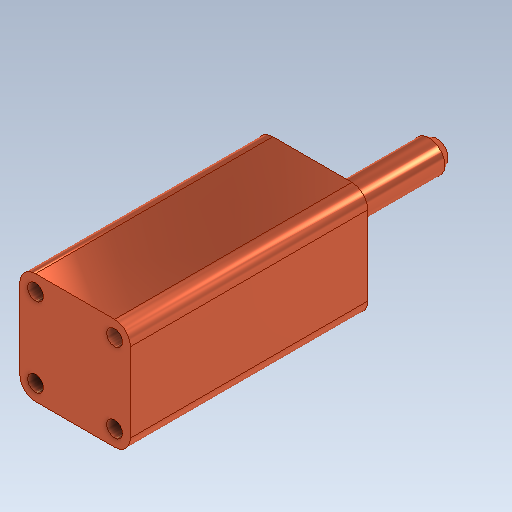
# Autodesk Inventor part: Silnik krokowy
Saved by Autodesk Inventor 2020 (Build 240168000, 168)
## iProperties
Created: 2021-10-14
Part Number: Silnik krokowy
Material: Ogólny
Document SubType Name: Modeling
Designer: Komputer
Density: 1 g/cm^3
Appearance: Gorący metal 1400F
Mass: 5.94241 g
Surface Area: 23.2204 cm^2
Volume: 5.94241 cm^3
Author: Komputer
Autodesk Inventor part; units mm, degrees
ref_plane "YZ Plane" through (0, 0, 0) normal (1, 0, 0) x (0, 1, 0)
ref_plane "XZ Plane" through (0, 0, 0) normal (0, 1, 0) x (-1, 0, 0)
ref_plane "XY Plane" through (0, 0, 0) normal (0, 0, 1) x (1, 0, 0)
sketch "Szkic1" plane through (0, 0, 0) normal (0, 0, 1) x (1, 0, 0)
  line L0 (7, -7) -> (-7, -7)
  line L1 (-7, -7) -> (-7, 7)
  line L2 (-7, 7) -> (7, 7)
  line L3 (7, 7) -> (7, -7)
  line L4 (7, -7) -> (-7, 7) construction
  line L5 (-7, -7) -> (7, 7) construction
  line L6 (0, 0) -> (-5.75, 0)
  line L7 (-7, 5.75) -> (-5, 5.75)
  line L8 (-5, 7) -> (-5, 5)
  line L9 (-5, 5) -> (5, 5)
  line L10 (5, 5) -> (5, -5)
  line L11 (5, -5) -> (-5, -5)
  line L12 (-5, -5) -> (-5, 5)
  circle A0 centre (-5, 5) radius 1
  circle A1 centre (5, 5) radius 1
  circle A2 centre (5, -5) radius 1
  circle A3 centre (-5, -5) radius 1
  circle A4 centre (0, 0) radius 5
  circle A5 centre (0, 0) radius 5.5
  circle A6 centre (0, 0) radius 2
  circle A7 centre (0, 0) radius 2.1
  dimension "d0" = 14
  dimension "d1" = 14
  dimension "d8" = 2
  dimension "d9" = 2
  dimension "d13" = 10
  dimension "d14" = 10
  dimension "d15" = 10
  dimension "d17" = 2
  dimension "d18" = 2
  dimension "d19" = 2
  dimension "d20" = 2
  dimension "d21" = 11
  dimension "d22" = 4
  dimension "d23" = 4.2
  constraints: 26 end point, 8 centre point, 8 coincident, 6 point on line, 3 perpendicular, 2 horizontal, 2 midpoint, 2 parallel
  measures "d0" distance of L1.end L2.end
  measures "d1" distance of L0.end L1.end
  measures "d8" distance of L7.start L7.end
  measures "d9" distance of L8.start L8.end
  measures "d13" distance of L8.end L9.end
  measures "d14" distance of L9.end L10.end
  measures "d15" distance of L10.end L11.end
  measures "d17" diameter of A0
  measures "d18" diameter of A1
  measures "d19" diameter of A2
  measures "d20" diameter of A3
  measures "d21" diameter of A5
  measures "d22" diameter of A6
  measures "d23" diameter of A7
extrude "Wyciągnięcie proste1" add sketch "Szkic1" along normal blind 30 contours L0 L1 L7 A0 L12 A5 A3 L11 A2 L10 A1 L9 L8 L2 L3 | L1 L2 L8 A0 L7 | A0 L9 A5 L12 | A5 L9 A4 L12 | L12 L6 A5 | A5 L9 | A6 | A7 | L12 A5 L6 | A4 L11 A5 L12 | A4 | L9 A5 L10 A4 | L9 A1 L10 A5 | A5 L11 A3 L12 | A4 L10 A5 L11 | L11 A5 | L10 A5 | A5 L10 A2 L11
sketch "Szkic2" plane through (0, 0, 0) normal (0, 0, -1) x (-1, 0, 0)
  line L0 (7, -7) -> (-7, -7)
  line L1 (-7, -7) -> (-7, 7)
  line L2 (-7, 7) -> (7, 7)
  line L3 (7, 7) -> (7, -7)
  line L4 (7, -7) -> (-7, 7) construction
  line L5 (-7, -7) -> (7, 7) construction
  line L6 (0, 0) -> (-5.75, 0)
  line L7 (-7, 5.75) -> (-5, 5.75)
  line L8 (-5, 7) -> (-5, 5)
  line L9 (-5, 5) -> (5, 5)
  line L10 (5, 5) -> (5, -5)
  line L11 (5, -5) -> (-5, -5)
  line L12 (-5, -5) -> (-5, 5)
  circle A0 centre (-5, 5) radius 1
  circle A1 centre (5, 5) radius 1
  circle A2 centre (5, -5) radius 1
  circle A3 centre (-5, -5) radius 1
  circle A4 centre (0, 0) radius 5
  circle A5 centre (0, 0) radius 5.5
  circle A6 centre (0, 0) radius 2
  circle A7 centre (0, 0) radius 2.1
  dimension "d26" = 14
  dimension "d27" = 14
  dimension "d28" = 2
  dimension "d29" = 2
  dimension "d30" = 10
  dimension "d31" = 10
  dimension "d32" = 10
  dimension "d33" = 2
  dimension "d34" = 2
  dimension "d35" = 2
  dimension "d36" = 2
  dimension "d37" = 11
  dimension "d38" = 4
  dimension "d39" = 4.2
  constraints: 26 end point, 8 centre point, 8 coincident, 6 point on line, 3 perpendicular, 2 horizontal, 2 midpoint, 2 parallel
  measures "d26" distance of L1.end L3.start
  measures "d27" distance of L0.end L1.end
  measures "d28" distance of L7.start L7.end
  measures "d29" distance of L8.start L12.end
  measures "d30" distance of L12.end L10.start
  measures "d31" distance of L10.start L11.start
  measures "d32" distance of L11.start L11.end
  measures "d33" diameter of A0
  measures "d34" diameter of A1
  measures "d35" diameter of A2
  measures "d36" diameter of A3
  measures "d37" diameter of A5
  measures "d38" diameter of A6
  measures "d39" diameter of A7
extrude "Wyciągnięcie proste2" add sketch "Szkic2" along normal blind 0.75 contours A6 | A7 | A4
fillet "Zaokrąglenie1" radius 2 4 edges at (-7, 7, 15) (7, 7, 15) (7, -7, 15) (-7, -7, 15)
fillet "Zaokrąglenie2" radius 0.5 1 edges at (5, 0, 0)
sketch "Szkic3" plane through (0, 0, -0.75) normal (0, 0, -1) x (-1, 0, 0)
  circle A0 centre (0, 0) radius 2
  dimension "d44" = 4
  constraints: 1 centre point, 1 coincident
  measures "d44" diameter of A0
extrude "Wyciągnięcie proste3" add sketch "Szkic3" along normal blind 15
chamfer "Faza1" distance 1 angle 30 1 edges at (2, 0, -15.75) measured on face at (-1.9935, -0.1609, -10.75)
sketch "Szkic4" plane through (0, 0, 0) normal (0, 0, -1) x (-1, 0, 0)
  circle A0 centre (-5, 5) radius 1 projected
  circle A1 centre (-5, 5) radius 1
  circle A2 centre (5, 5) radius 1 projected
  circle A3 centre (5, 5) radius 1
  circle A4 centre (5, -5) radius 1 projected
  circle A5 centre (5, -5) radius 1
  circle A6 centre (-5, -5) radius 1
  point P0 (0, 0)
  constraints: 4 centre point, 3 coincident
extrude "Wyciągnięcie proste4" add sketch "Szkic4" against normal blind 26.8
sketch "Szkic5" plane through (0, 0, 0) normal (0, 0, -1) x (-1, 0, 0)
  circle A0 centre (-5, 5) radius 1 projected
  circle A1 centre (-5, 5) radius 1
  circle A2 centre (5, 5) radius 1 projected
  circle A3 centre (5, 5) radius 1
  circle A4 centre (5, -5) radius 1 projected
  circle A5 centre (5, -5) radius 1
  circle A6 centre (-5, -5) radius 1 projected
  circle A7 centre (-5, -5) radius 1
  point P0 (0, 0)
  constraints: 4 centre point, 4 coincident
extrude "Wyciągnięcie proste5" cut sketch "Szkic5" against normal blind 3.2
